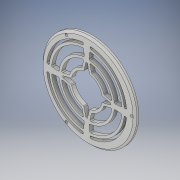
# Autodesk Inventor part: gimbalThrusterFrontCover
Saved by Autodesk Inventor 2018 (Build 220112000, 112)
## iProperties
Created: 2020-01-26
Part Number: gimbalThrusterFrontCover
Material: Generic
Document SubType Name: Modeling
Designer: anirudh
Density: 1 g/cm^3
Appearance: Default
Author: anirudh
Autodesk Inventor part; units mm, degrees
ref_plane "YZ Plane" through (0, 0, 0) normal (1, 0, 0) x (0, 1, 0)
ref_plane "XZ Plane" through (0, 0, 0) normal (0, 1, 0) x (-1, 0, 0)
ref_plane "XY Plane" through (0, 0, 0) normal (0, 0, 1) x (1, 0, 0)
sketch "Sketch2" plane through (0, 0, 0) normal (0, 0, 1) x (1, 0, 0)
  circle A0 centre (0, 0) radius 62.4586
  arc A1 (-0.568, 31.0918) -> (-3.0388, 31.0918) centre (-1.8034, 30.7975) ccw
  line L0 (-5.6134, 20.2828) -> (-3.0388, 31.0918)
  line L1 (2.0066, 20.2828) -> (-0.568, 31.0918)
  arc A2 (-32.8952, 1.2354) -> (-32.8952, -1.2354) centre (-32.6009, 0) ccw
  line L2 (-22.0862, -3.81) -> (-32.8952, -1.2354)
  line L3 (-22.0862, 3.81) -> (-32.8952, 1.2354)
  arc A3 (-3.0388, -31.0918) -> (-0.568, -31.0918) centre (-1.8034, -30.7975) ccw
  line L4 (2.0066, -20.2828) -> (-0.568, -31.0918)
  line L5 (-5.6134, -20.2828) -> (-3.0388, -31.0918)
  arc A4 (29.2884, -1.2354) -> (29.2884, 1.2354) centre (28.9941, 0) ccw
  line L6 (18.4794, 3.81) -> (29.2884, 1.2354)
  line L7 (18.4794, -3.81) -> (29.2884, -1.2354)
  arc A5 (-5.6134, 20.2828) -> (-22.0862, 3.81) centre (-1.8034, 0) ccw
  arc A6 (-22.0862, -3.81) -> (-5.6134, -20.2828) centre (-1.8034, 0) ccw
  arc A7 (2.0066, -20.2828) -> (18.4794, -3.81) centre (-1.8034, 0) ccw
  arc A8 (18.4794, 3.81) -> (2.0066, 20.2828) centre (-1.8034, 0) ccw
  dimension "d24" = 360
  constraints: 16 end point, 16 point on circle, 9 centre point, 1 coincident, 33 other
extrude "Extrusion2" add sketch "Sketch2" along normal blind 5.08
sketch "Sketch3" plane through (0, 0, 5.08) normal (0, 0, 1) x (1, 0, 0)
  circle A0 centre (0, 0) radius 62.4586 projected
  line L0 (0, 0) -> (57.8866, 0) construction
  circle A1 centre (-28.9433, 50.1313) radius 1.75
  circle A2 centre (-28.9433, -50.1313) radius 1.75
  circle A3 centre (57.8866, 0) radius 1.75
  dimension "d33" = 3.5
  dimension "d34" = 3.5
  dimension "d35" = 3.5
  constraints: 3 centre point, 2 end point, 1 coincident, 1 horizontal
  measures "d33" diameter of A1
  measures "d34" diameter of A2
  measures "d35" diameter of A3
extrude "Extrusion3" cut sketch "Sketch3" against normal blind 5.08 contours A1 | A2 | A3
sketch "Sketch5" plane through (0, 0, 5.08) normal (0, 0, 1) x (1, 0, 0)
  arc A0 (-5.6134, 20.2828) -> (-22.0862, 3.81) centre (-1.8034, 0) ccw projected
  arc A1 (-8.2482, 22.9238) -> (-24.7272, 6.4448) centre (-1.8034, 0) ccw
  arc A2 (-5.7085, 33.5862) -> (-35.3896, 3.9051) centre (-1.8034, 0) ccw
  line L0 (-24.7272, 6.4448) -> (-35.3896, 3.9051)
  line L1 (-8.2482, 22.9238) -> (-5.7085, 33.5862)
  line L2 (-1.8034, 0) -> (67.8238, 0) construction
  line L3 (-1.8034, 0) -> (66.1284, 0) construction
  line L4 (-51.775, 4.3719) -> (-54.9379, 4.6487)
  line L5 (-38.6502, 3.2237) -> (-48.6121, 4.0952)
  line L6 (-1.8034, 0) -> (67.0184, 0) construction
  line L7 (-1.8034, 0) -> (67.0184, 0) construction
  line L8 (-6.1753, 49.9716) -> (-6.4521, 53.1345)
  line L9 (-5.0271, 36.8468) -> (-5.8986, 46.8087)
  arc A3 (-5.0271, 36.8468) -> (-38.6502, 3.2237) centre (-1.8034, 0) ccw
  arc A4 (-5.8986, 46.8087) -> (-48.6121, 4.0952) centre (-1.8034, 0) ccw
  arc A5 (-6.1753, 49.9716) -> (-51.775, 4.3719) centre (-1.8034, 0) ccw
  arc A6 (-6.4521, 53.1345) -> (-54.9379, 4.6487) centre (-1.8034, 0) ccw
  line L10 (-8.2482, -22.9238) -> (-5.7085, -33.5862)
  line L11 (-6.1753, -49.9716) -> (-6.4521, -53.1345)
  line L12 (-5.0271, -36.8468) -> (-5.8986, -46.8087)
  arc A7 (-54.9379, -4.6487) -> (-6.4521, -53.1345) centre (-1.8034, 0) ccw
  arc A8 (-51.775, -4.3719) -> (-6.1753, -49.9716) centre (-1.8034, 0) ccw
  arc A9 (-48.6121, -4.0952) -> (-5.8986, -46.8087) centre (-1.8034, 0) ccw
  arc A10 (-38.6502, -3.2237) -> (-5.0271, -36.8468) centre (-1.8034, 0) ccw
  arc A11 (-35.3896, -3.9051) -> (-5.7085, -33.5862) centre (-1.8034, 0) ccw
  arc A12 (-24.7272, -6.4448) -> (-8.2482, -22.9238) centre (-1.8034, 0) ccw
  line L13 (-24.7272, -6.4448) -> (-35.3896, -3.9051)
  line L14 (-38.6502, -3.2237) -> (-48.6121, -4.0952)
  line L15 (-51.775, -4.3719) -> (-54.9379, -4.6487)
  line L16 (21.1204, -6.4448) -> (31.7828, -3.9051)
  line L17 (48.1682, -4.3719) -> (51.3311, -4.6487)
  line L18 (35.0434, -3.2237) -> (45.0053, -4.0952)
  arc A13 (2.8453, -53.1345) -> (51.3311, -4.6487) centre (-1.8034, 0) ccw
  arc A14 (2.5685, -49.9716) -> (48.1682, -4.3719) centre (-1.8034, 0) ccw
  arc A15 (2.2918, -46.8087) -> (45.0053, -4.0952) centre (-1.8034, 0) ccw
  arc A16 (1.4203, -36.8468) -> (35.0434, -3.2237) centre (-1.8034, 0) ccw
  arc A17 (2.1017, -33.5862) -> (31.7828, -3.9051) centre (-1.8034, 0) ccw
  arc A18 (4.6414, -22.9238) -> (21.1204, -6.4448) centre (-1.8034, 0) ccw
  line L19 (4.6414, -22.9238) -> (2.1017, -33.5862)
  line L20 (1.4203, -36.8468) -> (2.2918, -46.8087)
  line L21 (2.5685, -49.9716) -> (2.8453, -53.1345)
  line L22 (4.6414, 22.9238) -> (2.1017, 33.5862)
  line L23 (2.5685, 49.9716) -> (2.8453, 53.1345)
  line L24 (1.4203, 36.8468) -> (2.2918, 46.8087)
  arc A19 (51.3311, 4.6487) -> (2.8453, 53.1345) centre (-1.8034, 0) ccw
  arc A20 (48.1682, 4.3719) -> (2.5685, 49.9716) centre (-1.8034, 0) ccw
  arc A21 (45.0053, 4.0952) -> (2.2918, 46.8087) centre (-1.8034, 0) ccw
  arc A22 (35.0434, 3.2237) -> (1.4203, 36.8468) centre (-1.8034, 0) ccw
  arc A23 (31.7828, 3.9051) -> (2.1017, 33.5862) centre (-1.8034, 0) ccw
  arc A24 (21.1204, 6.4448) -> (4.6414, 22.9238) centre (-1.8034, 0) ccw
  line L25 (21.1204, 6.4448) -> (31.7828, 3.9051)
  line L26 (35.0434, 3.2237) -> (45.0053, 4.0952)
  line L27 (48.1682, 4.3719) -> (51.3311, 4.6487)
  point P0 (0, 0)
  point P1 (-32.8952, 1.2354)
  dimension "d89" = 360
  constraints: 56 end point, 48 point on circle, 24 centre point, 21 coincident, 4 horizontal, 121 other
extrude "Extrusion5" cut sketch "Sketch5" against normal blind 25.4
fillet "Fillet4" radius 1.27 56 edges at (-54.9379, 4.6487, 2.54) (-51.775, 4.3719, 2.54) (-6.4521, 53.1345, 2.54) (-6.1753, 49.9716, 2.54) (2.8453, 53.1345, 2.54) (2.5685, 49.9716, 2.54) (51.3311, 4.6487, 2.54) (48.1682, 4.3719, 2.54) (48.1682, -4.3719, 2.54) (51.3311, -4.6487, 2.54) (2.8453, -53.1345, 2.54) (2.5685, -49.9716, 2.54) (-6.4521, -53.1345, 2.54) (-6.1753, -49.9716, 2.54) (-54.9379, -4.6487, 2.54) (-51.775, -4.3719, 2.54) (-5.8986, 46.8087, 2.54) (-5.0271, 36.8468, 2.54) (-48.6121, 4.0952, 2.54) (-38.6502, 3.2237, 2.54) (-35.3896, 3.9051, 2.54) (-24.7272, 6.4448, 2.54) (-8.2482, 22.9238, 2.54) (-5.7085, 33.5862, 2.54) (2.1017, 33.5862, 2.54) (4.6414, 22.9238, 2.54) (21.1204, 6.4448, 2.54) (31.7828, 3.9051, 2.54) (35.0434, 3.2237, 2.54) (45.0053, 4.0952, 2.54) (1.4203, 36.8468, 2.54) (2.2918, 46.8087, 2.54) (-48.6121, -4.0952, 2.54) (-38.6502, -3.2237, 2.54) (-35.3896, -3.9051, 2.54) (-24.7272, -6.4448, 2.54) (-8.2482, -22.9238, 2.54) (-5.7085, -33.5862, 2.54) (-5.0271, -36.8468, 2.54) (-5.8986, -46.8087, 2.54) (2.2918, -46.8087, 2.54) (1.4203, -36.8468, 2.54) (2.1017, -33.5862, 2.54) (4.6414, -22.9238, 2.54) (35.0434, -3.2237, 2.54) (45.0053, -4.0952, 2.54) (21.1204, -6.4448, 2.54) (31.7828, -3.9051, 2.54) (-22.0862, -3.81, 2.54) (-22.0862, 3.81, 2.54) (-5.6134, -20.2828, 2.54) (2.0066, -20.2828, 2.54) (18.4794, -3.81, 2.54) (18.4794, 3.81, 2.54) (2.0066, 20.2828, 2.54) (-5.6134, 20.2828, 2.54)
chamfer "Chamfer1" distance 2.54 angle 45 1 edges at (-62.4586, 0, 5.08)
body "Solid2"
